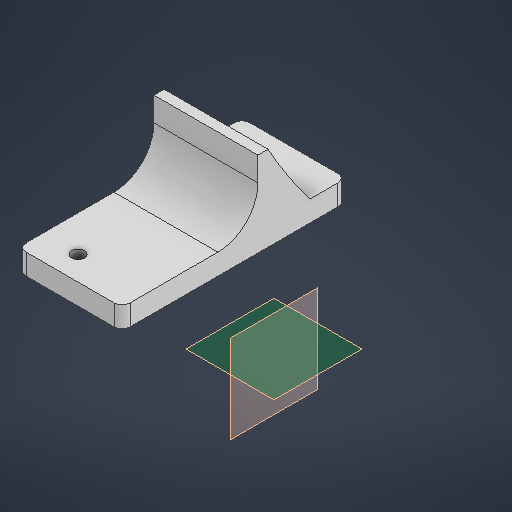
# Autodesk Inventor part: порожек
Saved by Autodesk Inventor 2026.2 (Build 302298000, 298)
## iProperties
Created: 2025-12-24
Part Number: порожек
Material: Типовые
Document SubType Name: Modeling
Designer: Phantom_HP2
Density: 1 g/cm^3
Appearance: По умолчанию
Author: Phantom_HP2
Autodesk Inventor part; units mm, degrees
ref_plane "YZ Plane" through (0, 0, 0) normal (1, 0, 0) x (0, 1, 0)
ref_plane "XZ Plane" through (0, 0, 0) normal (0, 1, 0) x (-1, 0, 0)
ref_plane "XY Plane" through (0, 0, 0) normal (0, 0, 1) x (1, 0, 0)
sketch "Эскиз1" plane through (0, 0, 0) normal (0, 1, 0) x (-1, 0, 0)
  line L0 (0, 0) -> (52, 0)
  line L1 (52, 0) -> (52, -56)
  line L2 (52, -56) -> (0, -56)
  line L3 (0, -56) -> (0, 0)
  dimension "d0" = 56
  dimension "d9" = 52
  constraints: 8 end point, 2 parallel, 1 horizontal, 1 perpendicular
  measures "d0" distance of L0.end L1.end
  measures "d9" distance of L1.end L2.end
extrude "Выдавливание1" add sketch "Эскиз1" along normal blind 5.2
ref_plane "РабПлоскость2" through (0, 3.2, -12) normal (0, -1, 0) x (1, 0, 0)
fillet "Сопряжение1" radius 2 4 edges at (0, 2.6, 0) (0, 2.6, -56) (-52, 2.6, -56) (-52, 2.6, 0)
ref_plane "РабПлоскость1" through (0, 0, -12) normal (1, 0, 0) x (0, 0, -1)
sketch "Эскиз4" plane through (0, 0, -12) normal (1, 0, 0) x (0, 0, -1)
  line L0 (34.9749, 5.2) -> (21.9749, 5.2)
  line L1 (21.9749, 21.2) -> (21.9749, 5.2)
  arc A0 (24.5222, 21.2) -> (34.9749, 5.2) centre (138.2876, 84.1082) ccw
  line L2 (21.9749, 21.2) -> (24.5222, 21.2)
  line L3 (44, 0) -> (44, 5.2) projected
  point P0 (-12, 0)
  dimension "d26" = 13
  dimension "d35" = 130
  dimension "d43" = 9.0251
  constraints: 6 end point, 2 point on circle, 1 centre point
  measures "d26" distance of L0.start L0.end
  measures "d35" radius of A0
  measures "d43" distance from line of L3 L0.start
extrude "Выдавливание4" add sketch "Эскиз4" against normal up to surface (52 mm away)
sketch "Эскиз5" plane through (0, 0, 0) normal (0, -1, 0) x (1, 0, 0)
  line L0 (0, 0) -> (-26, 0)
  line L1 (-26, 0) -> (-26, -56)
  line L2 (-26, -56) -> (0, -56)
  line L3 (0, -56) -> (0, 0)
  dimension "d37" = 26
  constraints: 8 end point, 2 parallel, 1 horizontal, 1 perpendicular
  measures "d37" distance of L2.end L1.end
extrude "Выдавливание5" cut sketch "Эскиз5" against normal blind 34
fillet "Сопряжение4" radius 2 2 edges at (-26, 2.6, 0) (-26, 2.6, -56)
fillet "Сопряжение5" radius 10 1 edges at (-39, 5.2, -33.9749)
sketch "Эскиз6" plane through (0, 5.2, 0) normal (0, 1, 0) x (1, 0, 0)
  circle A0 centre (-43, 6) radius 1.6
  circle A1 centre (-43, 50) radius 1.6
  line L0 (-52, 54) -> (-52, 46.9749) projected
  line L1 (-52, 23.9749) -> (-52, 2) projected
  line L2 (-50, 0) -> (-28, 0) projected
  line L3 (-28, 56) -> (-50, 56) projected
  point P0 (0, 0)
  dimension "d45" = 3.2
  dimension "d46" = 3.2
  dimension "d47" = 9
  dimension "d48" = 9
  dimension "d49" = 6
  dimension "d50" = 6
  constraints: 2 centre point
  measures "d45" diameter of A0
  measures "d46" diameter of A1
  measures "d47" distance from line of L0 A1.centre
  measures "d48" distance from line of L1 A0.centre
  measures "d49" distance from line of L2 A0.centre
  measures "d50" distance from line of L3 A1.centre
extrude "Выдавливание6" cut sketch "Эскиз6" against normal blind 40
